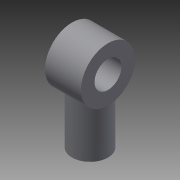
# Autodesk Inventor part: Floor Goal
Saved by Autodesk Inventor 2015 (Build 190159000, 159)
## iProperties
Created: 2016-12-01
Part Number: Floor Goal
Material: Generic
Document SubType Name: Modeling
Designer: Simms
Density: 1 g/cm^3
Appearance: Default
Author: Simms
Autodesk Inventor part; units mm, degrees
ref_plane "YZ Plane" through (0, 0, 0) normal (1, 0, 0) x (0, 1, 0)
ref_plane "XZ Plane" through (0, 0, 0) normal (0, 1, 0) x (-1, 0, 0)
ref_plane "XY Plane" through (0, 0, 0) normal (0, 0, 1) x (1, 0, 0)
sketch "Sketch1" plane through (0, 0, 0) normal (0, 1, 0) x (-1, 0, 0)
  circle A0 centre (0, 0) radius 6.35
  dimension "d0" = 12.7
  constraints: 1 centre point, 1 coincident
  measures "d0" diameter of A0
extrude "Extrusion1" add sketch "Sketch1" along normal blind 25.4
sketch "Sketch2" plane through (0, 0, 0) normal (1, 0, 0) x (0, 1, 0)
  line L0 (25.4, -6.35) -> (25.4, 6.35) projected
  circle A0 centre (25.4, 0) radius 9.525
  circle A1 centre (25.4, 0) radius 4.7625
  point P0 (0, 0)
  dimension "d3" = 19.05
  dimension "d4" = 9.525
  constraints: 2 centre point, 1 coincident, 1 midpoint
  measures "d3" diameter of A0
  measures "d4" diameter of A1
extrude "Extrusion2" cut sketch "Sketch2" along normal mid plane 25.4 contours A1 L0 | L0 A1 | A0
extrude "Extrusion3" add sketch "Sketch2" along normal mid plane 12.7
body "Solid1"
